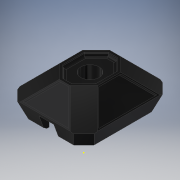
# Autodesk Inventor part: カメラ_外装
Saved by Autodesk Inventor 2018 (Build 220112000, 112)
## iProperties
Created: 2018-06-12
Part Number: カメラ_外装
Material: 一般
Document SubType Name: Modeling
Designer: taka
Density: 1 g/cm^3
Appearance: 滑らか - 黒
Mass: 52.2432 g
Surface Area: 167.376 cm^2
Volume: 52.2432 cm^3
Author: taka
Autodesk Inventor part; units mm, degrees
ref_plane "YZ Plane" through (0, 0, 0) normal (1, 0, 0) x (0, 1, 0)
ref_plane "XZ Plane" through (0, 0, 0) normal (0, 1, 0) x (-1, 0, 0)
ref_plane "XY Plane" through (0, 0, 0) normal (0, 0, 1) x (1, 0, 0)
sketch "スケッチ1" plane through (0, 0, 0) normal (0, 1, 0) x (-1, 0, 0)
  line L0 (0, 0) -> (52, 0)
  line L1 (52, 0) -> (52, -62)
  line L2 (52, -62) -> (0, -62)
  line L3 (0, -62) -> (0, 0)
  line L4 (38, -4) -> (14, -4)
  line L5 (4, -14) -> (4, -48)
  line L6 (14, -58) -> (38, -58)
  line L7 (48, -48) -> (48, -14)
  arc A0 (48, -14) -> (38, -4) centre (38, -14) ccw
  arc A1 (38, -58) -> (48, -48) centre (38, -48) ccw
  arc A2 (4, -48) -> (14, -58) centre (14, -48) ccw
  arc A3 (14, -4) -> (4, -14) centre (14, -14) ccw
  point P0 (4, -58)
  point P1 (4, -4)
  point P2 (48, -58)
  dimension "d0" = 52
  dimension "d1" = 62
  dimension "d2" = 44
  dimension "d3" = 54
  dimension "d4" = 4
  dimension "d5" = 4
  dimension "d6" = 10
  constraints: 16 end point, 8 point on circle, 8 tangent, 6 point on line, 4 centre point, 4 parallel, 3 equal radius, 2 horizontal, 2 perpendicular
  measures "d0" distance of L1.end L2.end
  measures "d1" distance of L0.end L1.end
  measures "d2" distance of point (48, -58) point (4, -58)
  measures "d3" distance of point (4, -58) point (4, -4)
  measures "d4" distance between parallel lines of L0 L4
  measures "d5" distance between parallel lines of L3 L5
  measures "d6" radius of A0
extrude "押し出し1" add sketch "スケッチ1" along normal blind 15
draft "面の勾配1" angle 20 pull direction (0, -1, 0) faces at (-17.333333, 5, 0) (-52, 10, -20.666667) (0, 10, -41.333333) (-34.666667, 5, -62) fixed edges at (-26, 0, 0) (-52, 0, -31) (0, 0, -31) (-26, 0, -62)
chamfer "面取り1" distance 8 angle 45 4 edges at (2.7298, 7.5, 2.7298) (2.7298, 7.5, -64.7298) (-54.7298, 7.5, -64.7298) (-54.7298, 7.5, 2.7298)
chamfer "面取り2" distance 2 angle 45 8 edges at (-52, 0, -31) (-47.7725, 0, -4.2275) (-26, 0, 0) (0, 0, -31) (-4.2275, 0, -57.7725) (-26, 0, -62) (-47.7725, 0, -57.7725) (-4.2275, 0, -4.2275)
sketch "スケッチ2" plane through (0, 15, 0) normal (0, 1, 0) x (1, 0, 0)
  line L0 (5.459554, 2.99542) -> (5.459554, 59.00458)
  line L1 (-2.99542, 67.459554) -> (-49.00458, 67.459554)
  line L2 (-57.459554, 59.00458) -> (-57.459554, 2.99542)
  line L3 (-49.00458, -5.459554) -> (-2.99542, -5.459554)
  line L4 (5.459554, 67.459554) -> (-57.459554, 67.459554)
  line L5 (-57.459554, 67.459554) -> (-57.459554, -5.459554)
  line L6 (-57.459554, -5.459554) -> (5.459554, -5.459554)
  line L7 (5.459554, -5.459554) -> (5.459554, 67.459554)
  point P0 (0, 0)
  constraints: 8 end point, 3 collinear, 2 parallel, 1 horizontal, 1 perpendicular, 1 point on line
extrude "押し出し2" add sketch "スケッチ2" along normal blind 16
draft "面の勾配3" angle 45 pull direction (0, 1, 0) faces at (5.459554, 25.666667, -40.33486) (-18.331807, 25.666667, 5.459554) (-57.459554, 25.666667, -21.66514) (-18.331807, 25.666667, -67.459554) fixed edges at (5.459554, 15, -31) (5.459554, 15, -63.232067) (5.459554, 15, 1.232067) (-53.232067, 15, 5.459554) (-26, 15, 5.459554) (1.232067, 15, 5.459554) (-57.459554, 15, -63.232067) (-57.459554, 15, -31) (-57.459554, 15, 1.232067) (1.232067, 15, -67.459554) (-26, 15, -67.459554) (-53.232067, 15, -67.459554)
chamfer "面取り3" distance 9 angle 45 4 edges at (-2.5404, 23, -59.4596) (-2.5404, 23, -2.5404) (-49.4596, 23, -2.5404) (-49.4596, 23, -59.4596)
sketch "スケッチ3" plane through (0, 31, 0) normal (0, 1, 0) x (1, 0, 0)
  line L0 (-21.56315, 51.459554) -> (-30.43685, 51.459554)
  line L1 (-41.459554, 40.43685) -> (-30.43685, 51.459554)
  line L2 (-41.459554, 40.43685) -> (-41.459554, 21.56315)
  line L3 (-30.43685, 10.540446) -> (-41.459554, 21.56315)
  line L4 (-30.43685, 10.540446) -> (-21.56315, 10.540446)
  line L5 (-10.540446, 21.56315) -> (-21.56315, 10.540446)
  line L6 (-10.540446, 21.56315) -> (-10.540446, 40.43685)
  line L7 (-21.56315, 51.459554) -> (-10.540446, 40.43685)
  line L8 (-21.56315, 51.459554) -> (-30.43685, 51.459554)
  circle A0 centre (-26, 31) radius 7.5
  point P0 (0, 0)
  dimension "d23" = 15
  dimension "d24" = 40.91911
  dimension "d25" = 30.91911
  dimension "d26" = 15.45955
  dimension "d27" = 20.45955
  constraints: 1 centre point
  measures "d23" diameter of A0
  measures "d24" distance between parallel lines of L4 L0
  measures "d25" distance between parallel lines of L2 L6
  measures "d26" distance from line of L6 A0.centre
  measures "d27" distance from line of A0.centre L4
extrude "押し出し3" cut sketch "スケッチ3" against normal through all contours A0
sketch "スケッチ4" plane through (0, 31, 0) normal (0, 1, 0) x (1, 0, 0)
  circle A0 centre (-26, 31) radius 7.5
  line L0 (-41.459554, 40.43685) -> (-30.43685, 51.459554)
  line L1 (-41.459554, 40.43685) -> (-41.459554, 21.56315)
  line L2 (-30.43685, 10.540446) -> (-41.459554, 21.56315)
  line L3 (-30.43685, 10.540446) -> (-21.56315, 10.540446)
  line L4 (-10.540446, 21.56315) -> (-21.56315, 10.540446)
  line L5 (-10.540446, 21.56315) -> (-10.540446, 40.43685)
  line L6 (-21.56315, 51.459554) -> (-10.540446, 40.43685)
  line L7 (-21.56315, 51.459554) -> (-30.43685, 51.459554)
  line L8 (-12.540446, 49.459554) -> (-39.459554, 49.459554)
  line L9 (-39.459554, 49.459554) -> (-39.459554, 12.540446)
  line L10 (-39.459554, 12.540446) -> (-12.540446, 12.540446)
  line L11 (-12.540446, 12.540446) -> (-12.540446, 49.459554)
  line L12 (-22.391577, 49.459554) -> (-12.540446, 39.608423)
  line L13 (-21.56315, 51.459554) -> (-10.540446, 40.43685)
  line L14 (-12.540446, 22.391577) -> (-22.391577, 12.540446)
  line L15 (-10.540446, 21.56315) -> (-21.56315, 10.540446)
  line L16 (-29.608423, 49.459554) -> (-39.459554, 39.608423)
  line L17 (-39.459554, 22.391577) -> (-29.608423, 12.540446)
  line L18 (-41.459554, 40.43685) -> (-30.43685, 51.459554)
  line L19 (-30.43685, 10.540446) -> (-41.459554, 21.56315)
  point P0 (0, 0)
  dimension "d30" = 2
  dimension "d31" = 2
  dimension "d33" = 2
  dimension "d34" = 2
  dimension "d35" = 2
  dimension "d36" = 2
  dimension "d37" = 2
  dimension "d38" = 2
  constraints: 16 end point, 8 point on line, 6 parallel, 1 horizontal, 1 perpendicular
  measures "d30" distance between parallel lines of L11 L5
  measures "d31" distance between parallel lines of L1 L9
  measures "d33" distance between parallel lines of L7 L8
  measures "d34" distance between parallel lines of L3 L10
  measures "d35" distance between parallel lines of L12 L6
  measures "d36" distance between parallel lines of L4 L14
  measures "d37" distance between parallel lines of L0 L16
  measures "d38" distance between parallel lines of L19 L17
extrude "押し出し4" cut sketch "スケッチ4" against normal blind 3 contours L16 L8 L12 L11 L14 L10 L17 L9
fillet "フィレット1" radius 2 8 edges at (-39.4596, 28, -31) (-34.534, 28, -44.534) (-26, 28, -49.4596) (-12.5404, 28, -31) (-17.466, 28, -44.534) (-17.466, 28, -17.466) (-34.534, 28, -17.466) (-26, 28, -12.5404)
sketch "スケッチ5" plane through (-57.459554, 15, -56.43685) normal (-0.7071068, 0.7071068, 0) x (-0.7071068, -0.7071068, 0)
  line L0 (-1, 48.941848) -> (-21.627417, 34.356061)
  line L1 (-21.627417, 34.356061) -> (-21.627417, 16.517638)
  line L2 (-21.627417, 16.517638) -> (-1, 1.931852)
  line L3 (-1, 1.931852) -> (-1, 48.941848)
  line L4 (0, 0) -> (-22.627417, 16)
  line L5 (0, 0) -> (0, 50.873699)
  line L6 (-22.627417, 34.873699) -> (0, 50.873699)
  line L7 (-22.627417, 16) -> (-22.627417, 34.873699)
  line L8 (0, 0) -> (0, 50.873699)
  point P0 (-30.023438, 56.43685)
  dimension "d51" = 1
  dimension "d52" = 1
  dimension "d53" = 1
  dimension "d54" = 1
  constraints: 8 end point, 5 parallel, 1 vertical
  measures "d51" distance between parallel lines of L6 L0
  measures "d52" distance between parallel lines of L5 L3
  measures "d53" distance between parallel lines of L4 L2
  measures "d54" distance between parallel lines of L7 L1
extrude "押し出し5" cut sketch "スケッチ5" against normal blind 2 contours L3 L2 L1 L0
sketch "スケッチ6" plane through (5.459554, 15, -56.43685) normal (0.7071068, 0.7071068, 0) x (-0.7071068, 0.7071068, 0)
  line L0 (21.627417, 34.356061) -> (21.627417, 16.517638)
  line L1 (21.627417, 16.517638) -> (1, 1.931852)
  line L2 (1, 1.931852) -> (1, 48.941848)
  line L3 (1, 48.941848) -> (21.627417, 34.356061)
  line L4 (22.627417, 34.873699) -> (22.627417, 16)
  line L5 (0, 50.873699) -> (22.627417, 34.873699)
  line L6 (22.627417, 16) -> (0, 0)
  line L7 (0, 50.873699) -> (0, 0)
  point P0 (-6.746114, 56.43685)
  dimension "d57" = 1
  dimension "d58" = 1
  dimension "d59" = 1
  dimension "d60" = 1
  constraints: 8 end point, 4 parallel, 1 vertical
  measures "d57" distance between parallel lines of L5 L3
  measures "d58" distance between parallel lines of L7 L2
  measures "d59" distance between parallel lines of L4 L0
  measures "d60" distance between parallel lines of L6 L1
extrude "押し出し6" cut sketch "スケッチ6" against normal blind 2 contours L0 L1 L2 L3
sketch "スケッチ7" plane through (-5.56315, 15, -67.459554) normal (0, 0.7071068, -0.7071068) x (-1, 0, 0)
  line L0 (24.356061, 21.627417) -> (16.517638, 21.627417)
  line L1 (16.517638, 21.627417) -> (1.931852, 1)
  line L2 (1.931852, 1) -> (38.941848, 1)
  line L3 (38.941848, 1) -> (24.356061, 21.627417)
  line L4 (24.873699, 22.627417) -> (40.873699, 0)
  line L5 (0, 0) -> (40.873699, 0)
  line L6 (0, 0) -> (16, 22.627417)
  line L7 (16, 22.627417) -> (24.873699, 22.627417)
  point P0 (-5.56315, 37.094506)
  dimension "d63" = 1
  dimension "d64" = 1
  dimension "d65" = 1
  dimension "d66" = 1
  constraints: 8 end point, 5 parallel, 1 horizontal
  measures "d63" distance between parallel lines of L7 L0
  measures "d64" distance between parallel lines of L4 L3
  measures "d65" distance between parallel lines of L5 L2
  measures "d66" distance between parallel lines of L6 L1
extrude "押し出し7" cut sketch "スケッチ7" against normal blind 2 contours L3 L2 L1 L0
sketch "スケッチ8" plane through (-46.43685, 15, 5.459554) normal (0, 0.7071068, 0.7071068) x (1, 0, 0)
  line L0 (1.931852, 1) -> (38.941848, 1)
  line L1 (38.941848, 1) -> (24.356061, 21.627417)
  line L2 (24.356061, 21.627417) -> (16.517638, 21.627417)
  line L3 (16.517638, 21.627417) -> (1.931852, 1)
  line L4 (0, 0) -> (16, 22.627417)
  line L5 (0, 0) -> (40.873699, 0)
  line L6 (16, 22.627417) -> (24.873699, 22.627417)
  line L7 (24.873699, 22.627417) -> (40.873699, 0)
  point P0 (46.43685, -6.746114)
  dimension "d69" = 1
  dimension "d70" = 1
  dimension "d71" = 1
  dimension "d72" = 1
  constraints: 8 end point, 5 parallel, 1 horizontal
  measures "d69" distance between parallel lines of L5 L0
  measures "d70" distance between parallel lines of L7 L1
  measures "d71" distance between parallel lines of L6 L2
  measures "d72" distance between parallel lines of L4 L3
extrude "押し出し8" cut sketch "スケッチ8" against normal blind 2 contours L3 L2 L1 L0
sketch "スケッチ9" plane through (0, 0, 0) normal (0, -1, 0) x (1, 0, 0)
  point P0 (0, 0)
sketch "スケッチ10" plane through (0, 15, 0) normal (0, -1, 0) x (1, 0, 0)
  circle A0 centre (-45, -41) radius 3
  circle A1 centre (-45, -21) radius 3
  circle A2 centre (-7, -41) radius 3
  circle A3 centre (-7, -21) radius 3
  line L0 (-38, -58) -> (-14, -58) projected
  line L1 (-48, -14) -> (-48, -48) projected
  line L2 (-4, -48) -> (-4, -14) projected
  line L3 (-45, -18) -> (-48, -18)
  line L4 (-45, -24) -> (-48, -24)
  line L5 (-4, -44) -> (-4, -38)
  line L6 (-4, -24) -> (-4, -18)
  line L7 (-48, -44) -> (-48, -38)
  line L8 (-48, -24) -> (-48, -18)
  line L9 (-45, -44) -> (-48, -44)
  line L10 (-48, -44) -> (-48, -38)
  line L11 (-45, -38) -> (-48, -38)
  line L12 (-45, -44) -> (-48, -44)
  line L13 (-48, -44) -> (-48, -38)
  line L14 (-48, -38) -> (-45, -38)
  line L15 (-45, -38) -> (-45, -44)
  line L16 (-48, -24) -> (-45, -24)
  line L17 (-45, -24) -> (-45, -18)
  line L18 (-45, -18) -> (-48, -18)
  line L19 (-48, -18) -> (-48, -24)
  line L20 (-7, -24) -> (-4, -24)
  line L21 (-4, -24) -> (-4, -18)
  line L22 (-4, -18) -> (-7, -18)
  line L23 (-7, -18) -> (-7, -24)
  line L24 (-7, -44) -> (-4, -44)
  line L25 (-4, -44) -> (-4, -38)
  line L26 (-4, -38) -> (-7, -38)
  line L27 (-7, -38) -> (-7, -44)
  point P0 (0, 0)
  dimension "d77" = 6
  dimension "d78" = 6
  dimension "d75" = 6
  dimension "d76" = 6
  dimension "d79" = 17
  dimension "d80" = 3
  dimension "d81" = 20
  dimension "d82" = 3
  dimension "d83" = 20
  dimension "d84" = 17
  dimension "d85" = 3
  dimension "d86" = 3
  constraints: 50 end point, 9 horizontal, 8 parallel, 7 perpendicular, 5 point on line, 4 collinear, 4 point on circle, 4 tangent, 2 centre point, 2 vertical alignment, 4 other
  measures "d75" diameter of A0
  measures "d76" diameter of A1
  measures "d79" distance from line of L0 A0.centre
  measures "d80" distance from line of L1 A0.centre
  measures "d81" distance of A1.centre A0.centre
  measures "d82" distance from line of L1 A1.centre
  measures "d83" distance of point (-7, -41) point (-7, -21)
  measures "d84" distance from line of L0 point (-7, -41)
  measures "d85" distance from line of L2 point (-7, -41)
  measures "d86" distance from line of L2 point (-7, -21)
extrude "押し出し9" add sketch "スケッチ10" along normal blind 15
sketch "スケッチ11" plane through (0, 0, 0) normal (0, -1, 0) x (1, 0, 0)
  arc A0 (-45, -44) -> (-45, -38) centre (-45, -41) ccw projected
  arc A1 (-45, -24) -> (-45, -18) centre (-45, -21) ccw projected
  arc A2 (-7, -18) -> (-7, -24) centre (-7, -21) ccw projected
  arc A3 (-7, -38) -> (-7, -44) centre (-7, -41) ccw projected
  circle A4 centre (-45, -41) radius 0.9
  circle A5 centre (-45, -21) radius 0.9
  circle A6 centre (-7, -41) radius 0.9
  circle A7 centre (-7, -21) radius 0.9
  point P0 (0, 0)
  dimension "d89" = 1.8
  dimension "d90" = 1.8
  dimension "d91" = 1.8
  dimension "d92" = 1.8
  constraints: 4 centre point, 4 coincident
  measures "d89" diameter of A4
  measures "d90" diameter of A5
  measures "d91" diameter of A6
  measures "d92" diameter of A7
extrude "押し出し10" cut sketch "スケッチ11" against normal blind 15
sketch "スケッチ12" plane through (0, 0, 0) normal (0, -1, 0) x (1, 0, 0)
  arc A0 (-48, -48) -> (-38, -58) centre (-38, -48) ccw
  line L0 (-48, -48) -> (-48, -44)
  arc A1 (-38, -4) -> (-48, -14) centre (-38, -14) ccw
  line L1 (-38, -4) -> (-14, -4)
  arc A2 (-4, -14) -> (-14, -4) centre (-14, -14) ccw
  line L2 (-4, -14) -> (-4, -18)
  arc A3 (-14, -58) -> (-4, -48) centre (-14, -48) ccw
  line L3 (-14, -58) -> (-38, -58)
  line L4 (-2, -9.283401) -> (-2, -52.716599)
  line L5 (-9.283401, -2) -> (-2, -9.283401)
  line L6 (-42.716599, -2) -> (-9.283401, -2)
  line L7 (-50, -9.283401) -> (-42.716599, -2)
  line L8 (-50, -52.716599) -> (-50, -9.283401)
  line L9 (-42.716599, -60) -> (-50, -52.716599)
  line L10 (-9.283401, -60) -> (-42.716599, -60)
  line L11 (-2, -52.716599) -> (-9.283401, -60)
  line L12 (-48, -44) -> (-4, -44)
  line L13 (-4, -44) -> (-4, -18)
  line L14 (-4, -18) -> (-48, -18)
  line L15 (-48, -18) -> (-48, -44)
  line L16 (-48, -44) -> (-45, -44)
  arc A4 (-45, -44) -> (-45, -38) centre (-45, -41) ccw
  line L17 (-45, -38) -> (-48, -38)
  line L18 (-48, -38) -> (-48, -24)
  line L19 (-48, -24) -> (-45, -24)
  arc A5 (-45, -24) -> (-45, -18) centre (-45, -21) ccw
  line L20 (-45, -18) -> (-48, -18)
  line L21 (-48, -18) -> (-48, -14)
  line L22 (-4, -18) -> (-7, -18)
  arc A6 (-7, -18) -> (-7, -24) centre (-7, -21) ccw
  line L23 (-7, -24) -> (-4, -24)
  line L24 (-4, -24) -> (-4, -38)
  line L25 (-4, -38) -> (-7, -38)
  arc A7 (-7, -38) -> (-7, -44) centre (-7, -41) ccw
  line L26 (-7, -44) -> (-4, -44)
  line L27 (-4, -44) -> (-4, -48)
  point P0 (0, 0)
  constraints: 8 end point, 2 parallel, 1 horizontal, 1 perpendicular
extrude "押し出し11" cut sketch "スケッチ12" against normal blind 3 contours L15 L17 A4 L12 | A4 L17 L15 L19 A5 L14 A6 L23 L13 L25 A7 L12 | A7 L25 L13 L12 | L15 L14 A5 L19 | L23 A6 L14 L13
sketch "スケッチ13" plane through (-14, 0, -4) normal (0, 0, -1) x (-1, 0, 0)
  line L0 (18, 0) -> (6, 0)
  line L1 (6, 0) -> (6, 12)
  line L2 (6, 12) -> (18, 12)
  line L3 (18, 12) -> (18, 0)
  line L4 (24, 0) -> (0, 0) projected
  line L5 (24, 0) -> (24, 15) projected
  point P0 (-14, 0)
  dimension "d97" = 12
  dimension "d98" = 12
  dimension "d99" = 24
  dimension "d100" = 6
  constraints: 8 end point, 2 parallel, 1 collinear, 1 horizontal, 1 perpendicular
  measures "d97" distance of L1.end L2.end
  measures "d98" distance of L0.end L1.end
  measures "d99" distance of L4.start L4.end
  measures "d100" distance between parallel lines of L5 L3
extrude "押し出し12" cut sketch "スケッチ13" along normal through all both and the other way through all
equation "\"d4\" = -0.5 * d3 + 0.5 * d1"
equation "\"d5\" = -0.5 * d2 + 0.5 * d0"
equation "\"d26\" = 0.5 * d25"
equation "\"d27\" = 0.5 * d24"
equation "\"d31\" = d30"
equation "\"d33\" = d30"
equation "\"d34\" = d30"
equation "\"d35\" = d30"
equation "\"d36\" = d30"
equation "\"d37\" = d30"
equation "\"d38\" = d30"
equation "\"d52\" = d51"
equation "\"d53\" = d51"
equation "\"d54\" = d51"
equation "\"d58\" = d57"
equation "\"d59\" = d57"
equation "\"d60\" = d57"
equation "\"d64\" = d63"
equation "\"d65\" = d63"
equation "\"d66\" = d63"
equation "\"d70\" = d69"
equation "\"d71\" = d69"
equation "\"d72\" = d69"
equation "\"d77\" = d75"
equation "\"d78\" = d75"
equation "\"d76\" = d75"
equation "\"d82\" = d80"
equation "\"d83\" = d81"
equation "\"d84\" = d79"
equation "\"d85\" = d80"
equation "\"d86\" = d80"
equation "\"d90\" = d89"
equation "\"d91\" = d89"
equation "\"d92\" = d89"
